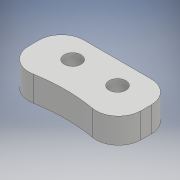
# Autodesk Inventor part: ruber
Saved by Autodesk Inventor 2018 (Build 220112000, 112)
## iProperties
Created: 2019-02-24
Part Number: ruber
Material: 一般
Document SubType Name: Modeling
Designer: kuwano
Density: 1 g/cm^3
Appearance: 既定
Author: kuwano
Autodesk Inventor part; units mm, degrees
ref_plane "YZ Plane" through (0, 0, 0) normal (1, 0, 0) x (0, 1, 0)
ref_plane "XZ Plane" through (0, 0, 0) normal (0, 1, 0) x (-1, 0, 0)
ref_plane "XY Plane" through (0, 0, 0) normal (0, 0, 1) x (1, 0, 0)
sketch "スケッチ1" plane through (0, 0, 0) normal (0, 0, 1) x (1, 0, 0)
  arc A0 (10, -1.7157) -> (-10, -1.7157) centre (0, -30) ccw
  line L0 (-10, -1.7157) -> (-10, 9.2843)
  line L1 (-10, 9.2843) -> (10, 9.2843)
  line L2 (10, 9.2843) -> (10, -1.7157)
  line L3 (-14, 0) -> (14, 0) projected
  point P0 (0, 0)
  point P1 (0, 0)
  dimension "d0" = 20
  dimension "d1" = 11
  dimension "d2" = 30
  constraints: 6 end point, 3 point on circle, 2 perpendicular, 1 centre point, 1 coincident, 1 tangent, 1 vertical
  measures "d0" distance of L0.end L1.end
  measures "d1" distance of L0.start L0.end
  measures "d2" radius of A0
extrude "押し出し1" add sketch "スケッチ1" along normal blind 4.5
fillet "フィレット1" radius 4 4 edges at (-10, 9.2843, 2.25) (10, 9.2843, 2.25) (10, -1.7157, 2.25) (-10, -1.7157, 2.25)
sketch "スケッチ2" plane through (0, 0, 4.5) normal (0, 0, 1) x (1, 0, 0)
  circle A0 centre (-4, 5.2843) radius 1.5
  circle A1 centre (4, 5.2843) radius 1.5
  line L0 (6, 9.2843) -> (-6, 9.2843) projected
  point P0 (0, 0)
  dimension "d7" = 3
  dimension "d8" = 3
  dimension "d9" = 4
  dimension "d10" = 4
  dimension "d11" = 4
  dimension "d12" = 4
  constraints: 2 centre point
  measures "d7" diameter of A0
  measures "d8" diameter of A1
  measures "d9" distance from line of L0 A0.centre
  measures "d10" distance from line of L0 A1.centre
  measures "d11" horizontal distance of point (0, 0) A0.centre
  measures "d12" horizontal distance of point (0, 0) A1.centre
extrude "押し出し2" cut sketch "スケッチ2" against normal blind 7.5
equation "\"d8\" = d7"
equation "\"d12\" = d11"
